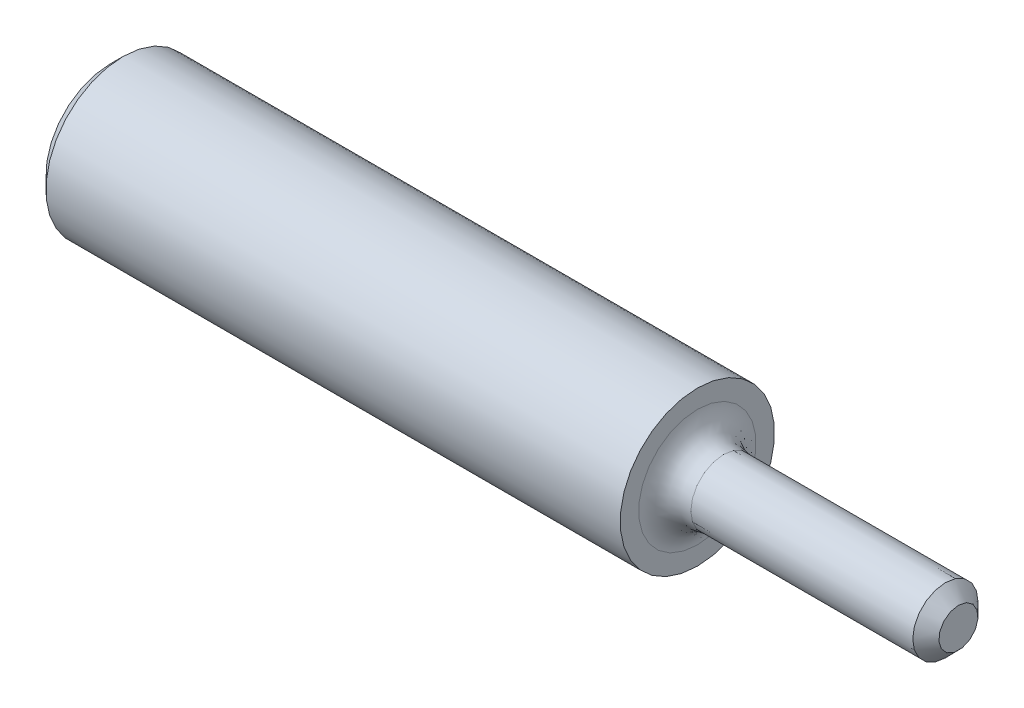
# Autodesk Inventor part: Shaft
Saved by Autodesk Inventor 2014 (Build 180170000, 170)
## iProperties
Created: 2014-08-25
Part Number: Shaft
Material: Steel
Document SubType Name: Modeling
Designer: sam
Density: 1 g/cm^3
Appearance: Steel
CustomPartVersion: 1
Author: sam
Autodesk Inventor part; units mm, degrees
ref_plane "Start Plane" through (0, 0, 0) normal (1, 0, 0) x (0, 1, 0)
ref_plane "XZ Plane" through (0, 0, 0) normal (0, 1, 0) x (-1, 0, 0)
ref_plane "XY Plane" through (0, 0, 0) normal (0, 0, 1) x (1, 0, 0)
sketch "Main Sketch" plane through (0, 0, 0) normal (0, 0, 1) x (1, 0, 0)
  line L0 (0, 0) -> (65, 0)
  line L1 (0, 0) -> (0, 5.912)
  line L2 (0, 5.912) -> (5, 5.912)
  line L3 (45, 5.912) -> (45, 2.5)
  line L4 (5, 5.912) -> (45, 5.912)
  line L5 (65, 2.5) -> (65, 0)
  line L6 (45, 2.5) -> (65, 2.5)
  dimension "d3" = 11.824
  dimension "d4" = 11.824
  dimension "d5" = 5
  constraints: 14 end point, 5 horizontal, 3 vertical
  measures "d3" diameter of L2 L0
  measures "d4" diameter of L4 L0
  measures "d5" diameter of L6 L0
revolve "Revolution1" add sketch "Main Sketch" angle 360 about axis through (0, 0, 0) along (1, 0, 0)
chamfer "Chamfer2" distance 1 angle 45 1 edges at (65, -2.5, 0) measured on face at (64.5, -2.5, 0)
chamfer "Chamfer1" distance 1 angle 45 1 edges at (0, -5.912, 0) measured on face at (0.5, -5.912, 0)
fillet "Fillet1" radius 2 1 edges at (45, -2.5, 0)
body "Solid1"
